Autodesk Inventor part; units mm, degrees
(part 2 of 3)
  spline S191 degree 2 poles (-31.6544, -13.3466) (-31.8311, -13.3678) (-32.0102, -13.4951) (-32.0102, -13.653) knots 0 0 0 1 2 2 2
  spline S192 degree 2 poles (-32.0102, -13.653) (-32.0102, -13.7684) (-31.8453, -13.9145) (-31.7063, -13.9145) knots 0 0 0 1 2 2 2
  spline S193 degree 2 poles (-31.7063, -13.9145) (-31.5178, -13.9145) (-31.2727, -13.6506) (-31.2727, -13.4503) knots 0 0 0 1 2 2 2
  line L231 (-31.2727, -13.4503) -> (-31.2727, -13.2925)
  spline S194 degree 2 poles (-29.3218, -12.7599) (-29.3948, -12.701) (-29.5362, -12.701) knots 0 0 0 1 1 1
  spline S195 degree 2 poles (-29.5362, -12.701) (-29.7176, -12.701) (-29.9627, -13.0309) (-29.9627, -13.3137) knots 0 0 0 1 2 2 2
  line L232 (-29.9627, -13.3137) -> (-29.9627, -14.1831)
  line L233 (-29.9627, -14.1831) -> (-30.3726, -14.1831)
  line L234 (-30.3726, -14.1831) -> (-30.3726, -12.3688)
  line L235 (-30.3726, -12.3688) -> (-29.9627, -12.3688)
  line L236 (-29.9627, -12.3688) -> (-29.9627, -12.7411)
  line L237 (-29.9627, -12.7411) -> (-29.9556, -12.7411)
  spline S196 degree 2 poles (-29.9556, -12.7411) (-29.8943, -12.5502) (-29.6446, -12.3358) (-29.4914, -12.3358) knots 0 0 0 1 2 2 2
  spline S197 degree 2 poles (-29.4914, -12.3358) (-29.3807, -12.3358) (-29.3218, -12.3688) knots 0 0 0 1 1 1
  line L238 (-29.3218, -12.3688) -> (-29.3218, -12.7599)
  line L239 (-28.6196, -14.1831) -> (-29.0296, -14.1831)
  line L240 (-29.0296, -14.1831) -> (-29.0296, -12.3688)
  line L241 (-29.0296, -12.3688) -> (-28.6196, -12.3688)
  line L242 (-28.6196, -12.3688) -> (-28.6196, -14.1831)
  spline S198 degree 2 poles (-28.8222, -11.9871) (-28.9236, -11.9871) (-29.0673, -11.8552) (-29.0673, -11.7538) knots 0 0 0 1 2 2 2
  spline S199 degree 2 poles (-29.0673, -11.7538) (-29.0673, -11.6525) (-28.9236, -11.5182) (-28.8222, -11.5182) knots 0 0 0 1 2 2 2
  spline S200 degree 2 poles (-28.8222, -11.5182) (-28.7186, -11.5182) (-28.5725, -11.6525) (-28.5725, -11.7538) knots 0 0 0 1 2 2 2
  spline S201 degree 2 poles (-28.5725, -11.7538) (-28.5725, -11.8504) (-28.7186, -11.9871) (-28.8222, -11.9871) knots 0 0 0 1 2 2 2
  line L243 (-27.6701, -14.1831) -> (-28.0824, -14.1831)
  line L244 (-28.0824, -14.1831) -> (-28.0824, -11.497)
  line L245 (-28.0824, -11.497) -> (-27.6701, -11.497)
  line L246 (-27.6701, -11.497) -> (-27.6701, -14.1831)
  line L247 (-26.7229, -14.1831) -> (-27.1352, -14.1831)
  line L248 (-27.1352, -14.1831) -> (-27.1352, -11.497)
  line L249 (-27.1352, -11.497) -> (-26.7229, -11.497)
  line L250 (-26.7229, -11.497) -> (-26.7229, -14.1831)
  line L251 (-24.7955, -14.1831) -> (-25.196, -14.1831)
  line L252 (-25.196, -14.1831) -> (-25.196, -13.9004)
  line L253 (-25.196, -13.9004) -> (-25.2031, -13.9004)
  spline S202 degree 2 poles (-25.2031, -13.9004) (-25.3892, -14.2255) (-25.7521, -14.2255) knots 0 0 0 1 1 1
  spline S203 degree 2 poles (-25.7521, -14.2255) (-26.0207, -14.2255) (-26.3247, -13.9357) (-26.3247, -13.6954) knots 0 0 0 1 2 2 2
  spline S204 degree 2 poles (-26.3247, -13.6954) (-26.3247, -13.1817) (-25.7309, -13.0969) knots 0 0 0 1 1 1
  line L254 (-25.7309, -13.0969) -> (-25.1937, -13.0215)
  spline S205 degree 2 poles (-25.1937, -13.0215) (-25.1937, -12.6327) (-25.5612, -12.6327) knots 0 0 0 1 1 1
  spline S206 degree 2 poles (-25.5612, -12.6327) (-25.8864, -12.6327) (-26.1456, -12.8566) knots 0 0 0 1 1 1
  line L255 (-26.1456, -12.8566) -> (-26.1456, -12.496)
  spline S207 degree 2 poles (-26.1456, -12.496) (-25.8605, -12.3264) (-25.4835, -12.3264) knots 0 0 0 1 1 1
  spline S208 degree 2 poles (-25.4835, -12.3264) (-24.7955, -12.3264) (-24.7955, -13.0026) knots 0 0 0 1 1 1
  line L256 (-24.7955, -13.0026) -> (-24.7955, -14.1831)
  line L257 (-25.1937, -13.2925) -> (-25.5754, -13.3466)
  spline S209 degree 2 poles (-25.5754, -13.3466) (-25.7521, -13.3678) (-25.9312, -13.4951) (-25.9312, -13.653) knots 0 0 0 1 2 2 2
  spline S210 degree 2 poles (-25.9312, -13.653) (-25.9312, -13.7684) (-25.7662, -13.9145) (-25.6272, -13.9145) knots 0 0 0 1 2 2 2
  spline S211 degree 2 poles (-25.6272, -13.9145) (-25.4387, -13.9145) (-25.1937, -13.6506) (-25.1937, -13.4503) knots 0 0 0 1 2 2 2
  line L258 (-25.1937, -13.4503) -> (-25.1937, -13.2925)
  line L259 (-21.8266, -14.1831) -> (-23.2522, -14.1831)
  line L260 (-23.2522, -14.1831) -> (-23.2522, -11.6431)
  line L261 (-23.2522, -11.6431) -> (-21.8832, -11.6431)
  line L262 (-21.8832, -11.6431) -> (-21.8832, -12.0012)
  line L263 (-21.8832, -12.0012) -> (-22.8304, -12.0012)
  line L264 (-22.8304, -12.0012) -> (-22.8304, -12.7199)
  line L265 (-22.8304, -12.7199) -> (-21.9562, -12.7199)
  line L266 (-21.9562, -12.7199) -> (-21.9562, -13.0757)
  line L267 (-21.9562, -13.0757) -> (-22.8304, -13.0757)
  line L268 (-22.8304, -13.0757) -> (-22.8304, -13.8273)
  line L269 (-22.8304, -13.8273) -> (-21.8266, -13.8273)
  line L270 (-21.8266, -13.8273) -> (-21.8266, -14.1831)
  line L271 (-21.5345, -14.1266) -> (-21.5345, -13.7472)
  spline S212 degree 2 poles (-21.5345, -13.7472) (-21.3036, -13.9216) (-21.0255, -13.9216) knots 0 0 0 1 1 1
  spline S213 degree 2 poles (-21.0255, -13.9216) (-20.6532, -13.9216) (-20.6532, -13.7001) knots 0 0 0 1 1 1
  spline S214 degree 2 poles (-20.6532, -13.7001) (-20.6532, -13.6388) (-20.7169, -13.5516) (-20.8252, -13.4857) (-20.9713, -13.4315) (-21.0632, -13.3985) knots 0 0 0 1 2 3 4 4 4
  spline S215 degree 2 poles (-21.0632, -13.3985) (-21.174, -13.3537) (-21.353, -13.2548) (-21.4709, -13.1299) (-21.5321, -12.9696) (-21.5321, -12.8636) knots 0 0 0 1 2 3 4 4 4
  spline S216 degree 2 poles (-21.5321, -12.8636) (-21.5321, -12.7317) (-21.4072, -12.5314) (-21.1975, -12.3947) (-20.9336, -12.3264) (-20.7923, -12.3264) knots 0 0 0 1 2 3 4 4 4
  spline S217 degree 2 poles (-20.7923, -12.3264) (-20.5401, -12.3264) (-20.3422, -12.4018) knots 0 0 0 1 1 1
  line L272 (-20.3422, -12.4018) -> (-20.3422, -12.7623)
  spline S218 degree 2 poles (-20.3422, -12.7623) (-20.5331, -12.6304) (-20.7805, -12.6304) knots 0 0 0 1 1 1
  spline S219 degree 2 poles (-20.7805, -12.6304) (-20.8582, -12.6304) (-20.9831, -12.6633) (-21.0727, -12.7199) (-21.1221, -12.8) (-21.1221, -12.8471) knots 0 0 0 1 2 3 4 4 4
  spline S220 degree 2 poles (-21.1221, -12.8471) (-21.1221, -12.906) (-21.0727, -12.9861) (-20.976, -13.0498) (-20.8394, -13.1016) (-20.7499, -13.1299) knots 0 0 0 1 2 3 4 4 4
  spline S221 degree 2 poles (-20.7499, -13.1299) (-20.6344, -13.1794) (-20.4483, -13.2783) (-20.3163, -13.4032) (-20.2456, -13.5681) (-20.2456, -13.6812) knots 0 0 0 1 2 3 4 4 4
  spline S222 degree 2 poles (-20.2456, -13.6812) (-20.2456, -13.8202) (-20.3729, -14.0252) (-20.5849, -14.1595) (-20.8629, -14.2255) (-21.0185, -14.2255) knots 0 0 0 1 2 3 4 4 4
  spline S223 degree 2 poles (-21.0185, -14.2255) (-21.3153, -14.2255) (-21.5345, -14.1266) knots 0 0 0 1 1 1
  spline S224 degree 2 poles (-18.8979, -14.1619) (-19.0204, -14.2232) (-19.216, -14.2232) knots 0 0 0 1 1 1
  spline S225 degree 2 poles (-19.216, -14.2232) (-19.7437, -14.2232) (-19.7437, -13.7166) knots 0 0 0 1 1 1
  line L273 (-19.7437, -13.7166) -> (-19.7437, -12.6916)
  line L274 (-19.7437, -12.6916) -> (-20.0477, -12.6916)
  line L275 (-20.0477, -12.6916) -> (-20.0477, -12.3688)
  line L276 (-20.0477, -12.3688) -> (-19.7437, -12.3688)
  line L277 (-19.7437, -12.3688) -> (-19.7437, -11.9494)
  line L278 (-19.7437, -11.9494) -> (-19.3338, -11.8316)
  line L279 (-19.3338, -11.8316) -> (-19.3338, -12.3688)
  line L280 (-19.3338, -12.3688) -> (-18.8979, -12.3688)
  line L281 (-18.8979, -12.3688) -> (-18.8979, -12.6916)
  line L282 (-18.8979, -12.6916) -> (-19.3338, -12.6916)
  line L283 (-19.3338, -12.6916) -> (-19.3338, -13.5988)
  spline S226 degree 2 poles (-19.3338, -13.5988) (-19.3338, -13.759) (-19.216, -13.898) (-19.0793, -13.898) knots 0 0 0 1 2 2 2
  spline S227 degree 2 poles (-19.0793, -13.898) (-18.9756, -13.898) (-18.8979, -13.8367) knots 0 0 0 1 1 1
  line L284 (-18.8979, -13.8367) -> (-18.8979, -14.1619)
  line L285 (-18.1345, -14.1831) -> (-18.5444, -14.1831)
  line L286 (-18.5444, -14.1831) -> (-18.5444, -12.3688)
  line L287 (-18.5444, -12.3688) -> (-18.1345, -12.3688)
  line L288 (-18.1345, -12.3688) -> (-18.1345, -14.1831)
  spline S228 degree 2 poles (-18.3371, -11.9871) (-18.4384, -11.9871) (-18.5821, -11.8552) (-18.5821, -11.7538) knots 0 0 0 1 2 2 2
  spline S229 degree 2 poles (-18.5821, -11.7538) (-18.5821, -11.6525) (-18.4384, -11.5182) (-18.3371, -11.5182) knots 0 0 0 1 2 2 2
  spline S230 degree 2 poles (-18.3371, -11.5182) (-18.2334, -11.5182) (-18.0873, -11.6525) (-18.0873, -11.7538) knots 0 0 0 1 2 2 2
  spline S231 degree 2 poles (-18.0873, -11.7538) (-18.0873, -11.8504) (-18.2334, -11.9871) (-18.3371, -11.9871) knots 0 0 0 1 2 2 2
  line L289 (-14.8852, -14.1831) -> (-15.2952, -14.1831)
  line L290 (-15.2952, -14.1831) -> (-15.2952, -13.1935)
  spline S232 degree 2 poles (-15.2952, -13.1935) (-15.2952, -12.9084) (-15.4578, -12.6539) (-15.6486, -12.6539) knots 0 0 0 1 2 2 2
  spline S233 degree 2 poles (-15.6486, -12.6539) (-15.8089, -12.6539) (-16.0351, -12.9767) (-16.0351, -13.2006) knots 0 0 0 1 2 2 2
  line L291 (-16.0351, -13.2006) -> (-16.0351, -14.1831)
  line L292 (-16.0351, -14.1831) -> (-16.4474, -14.1831)
  line L293 (-16.4474, -14.1831) -> (-16.4474, -13.1605)
  spline S234 degree 2 poles (-16.4474, -13.1605) (-16.4474, -12.6539) (-16.8055, -12.6539) knots 0 0 0 1 1 1
  spline S235 degree 2 poles (-16.8055, -12.6539) (-16.9728, -12.6539) (-17.1873, -12.9579) (-17.1873, -13.2006) knots 0 0 0 1 2 2 2
  line L294 (-17.1873, -13.2006) -> (-17.1873, -14.1831)
  line L295 (-17.1873, -14.1831) -> (-17.5972, -14.1831)
  line L296 (-17.5972, -14.1831) -> (-17.5972, -12.3688)
  line L297 (-17.5972, -12.3688) -> (-17.1873, -12.3688)
  line L298 (-17.1873, -12.3688) -> (-17.1873, -12.6563)
  line L299 (-17.1873, -12.6563) -> (-17.1802, -12.6563)
  spline S236 degree 2 poles (-17.1802, -12.6563) (-16.9823, -12.3264) (-16.6076, -12.3264) knots 0 0 0 1 1 1
  spline S237 degree 2 poles (-16.6076, -12.3264) (-16.4191, -12.3264) (-16.1387, -12.5337) (-16.0869, -12.701) knots 0 0 0 1 2 2 2
  spline S238 degree 2 poles (-16.0869, -12.701) (-15.8843, -12.3264) (-15.4837, -12.3264) knots 0 0 0 1 1 1
  spline S239 degree 2 poles (-15.4837, -12.3264) (-14.8852, -12.3264) (-14.8852, -13.0663) knots 0 0 0 1 1 1
  line L300 (-14.8852, -13.0663) -> (-14.8852, -14.1831)
  line L301 (-12.8023, -14.1831) -> (-13.2123, -14.1831)
  line L302 (-13.2123, -14.1831) -> (-13.2123, -13.8956)
  line L303 (-13.2123, -13.8956) -> (-13.2194, -13.8956)
  spline S240 degree 2 poles (-13.2194, -13.8956) (-13.3985, -14.2255) (-13.7778, -14.2255) knots 0 0 0 1 1 1
  spline S241 degree 2 poles (-13.7778, -14.2255) (-14.4187, -14.2255) (-14.4187, -13.4527) knots 0 0 0 1 1 1
  line L304 (-14.4187, -13.4527) -> (-14.4187, -12.3688)
  line L305 (-14.4187, -12.3688) -> (-14.0087, -12.3688)
  line L306 (-14.0087, -12.3688) -> (-14.0087, -13.4103)
  spline S242 degree 2 poles (-14.0087, -13.4103) (-14.0087, -13.9004) (-13.6317, -13.9004) knots 0 0 0 1 1 1
  spline S243 degree 2 poles (-13.6317, -13.9004) (-13.4479, -13.9004) (-13.2123, -13.6317) (-13.2123, -13.4126) knots 0 0 0 1 2 2 2
  line L307 (-13.2123, -13.4126) -> (-13.2123, -12.3688)
  line L308 (-13.2123, -12.3688) -> (-12.8023, -12.3688)
  line L309 (-12.8023, -12.3688) -> (-12.8023, -14.1831)
  line L310 (-11.8528, -14.1831) -> (-12.2651, -14.1831)
  line L311 (-12.2651, -14.1831) -> (-12.2651, -11.497)
  line L312 (-12.2651, -11.497) -> (-11.8528, -11.497)
  line L313 (-11.8528, -11.497) -> (-11.8528, -14.1831)
  line L314 (-9.9254, -14.1831) -> (-10.326, -14.1831)
  line L315 (-10.326, -14.1831) -> (-10.326, -13.9004)
  line L316 (-10.326, -13.9004) -> (-10.333, -13.9004)
  spline S244 degree 2 poles (-10.333, -13.9004) (-10.5192, -14.2255) (-10.882, -14.2255) knots 0 0 0 1 1 1
  spline S245 degree 2 poles (-10.882, -14.2255) (-11.1506, -14.2255) (-11.4546, -13.9357) (-11.4546, -13.6954) knots 0 0 0 1 2 2 2
  spline S246 degree 2 poles (-11.4546, -13.6954) (-11.4546, -13.1817) (-10.8608, -13.0969) knots 0 0 0 1 1 1
  line L317 (-10.8608, -13.0969) -> (-10.3236, -13.0215)
  spline S247 degree 2 poles (-10.3236, -13.0215) (-10.3236, -12.6327) (-10.6912, -12.6327) knots 0 0 0 1 1 1
  spline S248 degree 2 poles (-10.6912, -12.6327) (-11.0163, -12.6327) (-11.2755, -12.8566) knots 0 0 0 1 1 1
  line L318 (-11.2755, -12.8566) -> (-11.2755, -12.496)
  spline S249 degree 2 poles (-11.2755, -12.496) (-10.9904, -12.3264) (-10.6134, -12.3264) knots 0 0 0 1 1 1
  spline S250 degree 2 poles (-10.6134, -12.3264) (-9.9254, -12.3264) (-9.9254, -13.0026) knots 0 0 0 1 1 1
  line L319 (-9.9254, -13.0026) -> (-9.9254, -14.1831)
  line L320 (-10.3236, -13.2925) -> (-10.7053, -13.3466)
  spline S251 degree 2 poles (-10.7053, -13.3466) (-10.882, -13.3678) (-11.0611, -13.4951) (-11.0611, -13.653) knots 0 0 0 1 2 2 2
  spline S252 degree 2 poles (-11.0611, -13.653) (-11.0611, -13.7684) (-10.8962, -13.9145) (-10.7571, -13.9145) knots 0 0 0 1 2 2 2
  spline S253 degree 2 poles (-10.7571, -13.9145) (-10.5686, -13.9145) (-10.3236, -13.6506) (-10.3236, -13.4503) knots 0 0 0 1 2 2 2
  line L321 (-10.3236, -13.4503) -> (-10.3236, -13.2925)
  line L322 (-7.7742, -14.1831) -> (-8.1865, -14.1831)
  line L323 (-8.1865, -14.1831) -> (-8.1865, -13.8744)
  line L324 (-8.1865, -13.8744) -> (-8.1936, -13.8744)
  spline S254 degree 2 poles (-8.1936, -13.8744) (-8.3915, -14.2255) (-8.8038, -14.2255) knots 0 0 0 1 1 1
  spline S255 degree 2 poles (-8.8038, -14.2255) (-9.1384, -14.2255) (-9.5413, -13.7378) (-9.5413, -13.3184) knots 0 0 0 1 2 2 2
  spline S256 degree 2 poles (-9.5413, -13.3184) (-9.5413, -12.8683) (-9.096, -12.3264) (-8.7261, -12.3264) knots 0 0 0 1 2 2 2
  spline S257 degree 2 poles (-8.7261, -12.3264) (-8.3609, -12.3264) (-8.1936, -12.6209) knots 0 0 0 1 1 1
  line L325 (-8.1936, -12.6209) -> (-8.1865, -12.6209)
  line L326 (-8.1865, -12.6209) -> (-8.1865, -11.497)
  line L327 (-8.1865, -11.497) -> (-7.7742, -11.497)
  line L328 (-7.7742, -11.497) -> (-7.7742, -14.1831)
  line L329 (-8.1818, -13.3537) -> (-8.1818, -13.1157)
  spline S258 degree 2 poles (-8.1818, -13.1157) (-8.1818, -12.9225) (-8.4316, -12.6539) (-8.6271, -12.6539) knots 0 0 0 1 2 2 2
  spline S259 degree 2 poles (-8.6271, -12.6539) (-8.858, -12.6539) (-9.1219, -12.9979) (-9.1219, -13.3019) knots 0 0 0 1 2 2 2
  spline S260 degree 2 poles (-9.1219, -13.3019) (-9.1219, -13.5799) (-8.8675, -13.9004) (-8.653, -13.9004) knots 0 0 0 1 2 2 2
  spline S261 degree 2 poles (-8.653, -13.9004) (-8.4433, -13.9004) (-8.1818, -13.5893) (-8.1818, -13.3537) knots 0 0 0 1 2 2 2
  spline S262 degree 2 poles (-6.4335, -14.2255) (-6.8529, -14.2255) (-7.3548, -13.7166) (-7.3548, -13.2972) knots 0 0 0 1 2 2 2
  spline S263 degree 2 poles (-7.3548, -13.2972) (-7.3548, -12.8401) (-6.8317, -12.3264) (-6.3887, -12.3264) knots 0 0 0 1 2 2 2
  spline S264 degree 2 poles (-6.3887, -12.3264) (-5.9646, -12.3264) (-5.4886, -12.8259) (-5.4886, -13.2689) knots 0 0 0 1 2 2 2
  spline S265 degree 2 poles (-5.4886, -13.2689) (-5.4886, -13.7024) (-6.0023, -14.2255) (-6.4335, -14.2255) knots 0 0 0 1 2 2 2
  spline S266 degree 2 poles (-6.4146, -12.6539) (-6.655, -12.6539) (-6.9354, -12.9909) (-6.9354, -13.2877) knots 0 0 0 1 2 2 2
  spline S267 degree 2 poles (-6.9354, -13.2877) (-6.9354, -13.5728) (-6.6526, -13.9004) (-6.4146, -13.9004) knots 0 0 0 1 2 2 2
  spline S268 degree 2 poles (-6.4146, -13.9004) (-6.1719, -13.9004) (-5.9104, -13.5776) (-5.9104, -13.2807) knots 0 0 0 1 2 2 2
  spline S269 degree 2 poles (-5.9104, -13.2807) (-5.9104, -12.9791) (-6.1719, -12.6539) (-6.4146, -12.6539) knots 0 0 0 1 2 2 2
  spline S270 degree 2 poles (-4.0184, -12.7599) (-4.0914, -12.701) (-4.2328, -12.701) knots 0 0 0 1 1 1
  spline S271 degree 2 poles (-4.2328, -12.701) (-4.4142, -12.701) (-4.6593, -13.0309) (-4.6593, -13.3137) knots 0 0 0 1 2 2 2
  line L330 (-4.6593, -13.3137) -> (-4.6593, -14.1831)
  line L331 (-4.6593, -14.1831) -> (-5.0692, -14.1831)
  line L332 (-5.0692, -14.1831) -> (-5.0692, -12.3688)
  line L333 (-5.0692, -12.3688) -> (-4.6593, -12.3688)
  line L334 (-4.6593, -12.3688) -> (-4.6593, -12.7411)
  line L335 (-4.6593, -12.7411) -> (-4.6522, -12.7411)
  spline S272 degree 2 poles (-4.6522, -12.7411) (-4.5909, -12.5502) (-4.3412, -12.3358) (-4.188, -12.3358) knots 0 0 0 1 2 2 2
  spline S273 degree 2 poles (-4.188, -12.3358) (-4.0773, -12.3358) (-4.0184, -12.3688) knots 0 0 0 1 1 1
  line L336 (-4.0184, -12.3688) -> (-4.0184, -12.7599)
  line L337 (-2.3337, -14.1831) -> (-2.7342, -14.1831)
  line L338 (-2.7342, -14.1831) -> (-2.7342, -13.9004)
  line L339 (-2.7342, -13.9004) -> (-2.7413, -13.9004)
  spline S274 degree 2 poles (-2.7413, -13.9004) (-2.9274, -14.2255) (-3.2903, -14.2255) knots 0 0 0 1 1 1
  spline S275 degree 2 poles (-3.2903, -14.2255) (-3.5589, -14.2255) (-3.8629, -13.9357) (-3.8629, -13.6954) knots 0 0 0 1 2 2 2
  spline S276 degree 2 poles (-3.8629, -13.6954) (-3.8629, -13.1817) (-3.2691, -13.0969) knots 0 0 0 1 1 1
  line L340 (-3.2691, -13.0969) -> (-2.7319, -13.0215)
  spline S277 degree 2 poles (-2.7319, -13.0215) (-2.7319, -12.6327) (-3.0994, -12.6327) knots 0 0 0 1 1 1
  spline S278 degree 2 poles (-3.0994, -12.6327) (-3.4246, -12.6327) (-3.6838, -12.8566) knots 0 0 0 1 1 1
  line L341 (-3.6838, -12.8566) -> (-3.6838, -12.496)
  spline S279 degree 2 poles (-3.6838, -12.496) (-3.3987, -12.3264) (-3.0217, -12.3264) knots 0 0 0 1 1 1
  spline S280 degree 2 poles (-3.0217, -12.3264) (-2.3337, -12.3264) (-2.3337, -13.0026) knots 0 0 0 1 1 1
  line L342 (-2.3337, -13.0026) -> (-2.3337, -14.1831)
  line L343 (-2.7319, -13.2925) -> (-3.1136, -13.3466)
  spline S281 degree 2 poles (-3.1136, -13.3466) (-3.2903, -13.3678) (-3.4694, -13.4951) (-3.4694, -13.653) knots 0 0 0 1 2 2 2
  spline S282 degree 2 poles (-3.4694, -13.653) (-3.4694, -13.7684) (-3.3044, -13.9145) (-3.1654, -13.9145) knots 0 0 0 1 2 2 2
  spline S283 degree 2 poles (-3.1654, -13.9145) (-2.9769, -13.9145) (-2.7319, -13.6506) (-2.7319, -13.4503) knots 0 0 0 1 2 2 2
  line L344 (-2.7319, -13.4503) -> (-2.7319, -13.2925)
  line L345 (1.2007, -11.6431) -> (0.2888, -14.1831)
  line L346 (0.2888, -14.1831) -> (-0.1824, -14.1831)
  line L347 (-0.1824, -14.1831) -> (-1.0778, -11.6431)
  line L348 (-1.0778, -11.6431) -> (-0.6183, -11.6431)
  line L349 (-0.6183, -11.6431) -> (0.0084, -13.5705)
  spline S284 degree 2 poles (0.0084, -13.5705) (0.039, -13.6624) (0.0555, -13.7849) knots 0 0 0 1 1 1
  line L350 (0.0555, -13.7849) -> (0.0626, -13.7849)
  spline S285 degree 2 poles (0.0626, -13.7849) (0.0744, -13.6836) (0.1144, -13.5658) knots 0 0 0 1 1 1
  line L351 (0.1144, -13.5658) -> (0.7553, -11.6431)
  line L352 (0.7553, -11.6431) -> (1.2007, -11.6431)
  line L353 (3.6912, -14.1831) -> (3.2317, -14.1831)
  line L354 (3.2317, -14.1831) -> (2.0183, -12.317)
  spline S286 degree 2 poles (2.0183, -12.317) (1.9711, -12.2463) (1.9429, -12.1685) knots 0 0 0 1 1 1
  line L355 (1.9429, -12.1685) -> (1.9311, -12.1685)
  spline S287 degree 2 poles (1.9311, -12.1685) (1.9452, -12.251) (1.9452, -12.5173) knots 0 0 0 1 1 1
  line L356 (1.9452, -12.5173) -> (1.9452, -14.1831)
  line L357 (1.9452, -14.1831) -> (1.5376, -14.1831)
  line L358 (1.5376, -14.1831) -> (1.5376, -11.6431)
  line L359 (1.5376, -11.6431) -> (2.0277, -11.6431)
  line L360 (2.0277, -11.6431) -> (3.2011, -13.4668)
  spline S288 degree 2 poles (3.2011, -13.4668) (3.2765, -13.5799) (3.2977, -13.6223) knots 0 0 0 1 1 1
  line L361 (3.2977, -13.6223) -> (3.3048, -13.6223)
  spline S289 degree 2 poles (3.3048, -13.6223) (3.2859, -13.521) (3.2859, -13.2807) knots 0 0 0 1 1 1
  line L362 (3.2859, -13.2807) -> (3.2859, -11.6431)
  line L363 (3.2859, -11.6431) -> (3.6912, -11.6431)
  line L364 (3.6912, -11.6431) -> (3.6912, -14.1831)
  line L365 (4.2025, -14.0818) -> (4.2025, -13.6482)
  spline S290 degree 2 poles (4.2025, -13.6482) (4.2614, -13.7024) (4.424, -13.7873) (4.603, -13.8438) (4.7845, -13.8768) (4.8599, -13.8768) knots 0 0 0 1 2 3 4 4 4
  spline S291 degree 2 poles (4.8599, -13.8768) (5.1261, -13.8768) (5.3876, -13.7001) (5.3876, -13.5304) knots 0 0 0 1 2 2 2
  spline S292 degree 2 poles (5.3876, -13.5304) (5.3876, -13.4409) (5.3005, -13.3089) (5.145, -13.1982) (4.9329, -13.0969) (4.8127, -13.0427) knots 0 0 0 1 2 3 4 4 4
  spline S293 degree 2 poles (4.8127, -13.0427) (4.6831, -12.9744) (4.4617, -12.8306) (4.2967, -12.661) (4.2025, -12.4442) (4.2025, -12.2981) knots 0 0 0 1 2 3 4 4 4
  spline S294 degree 2 poles (4.2025, -12.2981) (4.2025, -12.1191) (4.3627, -11.8552) (4.6266, -11.6832) (4.9635, -11.6007) (5.1402, -11.6007) knots 0 0 0 1 2 3 4 4 4
  spline S295 degree 2 poles (5.1402, -11.6007) (5.5384, -11.6007) (5.7199, -11.6902) knots 0 0 0 1 1 1
  line L366 (5.7199, -11.6902) -> (5.7199, -12.1073)
  spline S296 degree 2 poles (5.7199, -12.1073) (5.5031, -11.9518) (5.1638, -11.9518) knots 0 0 0 1 1 1
  spline S297 degree 2 poles (5.1638, -11.9518) (5.0696, -11.9518) (4.8834, -11.9871) (4.7373, -12.0696) (4.6454, -12.1968) (4.6454, -12.2863) knots 0 0 0 1 2 3 4 4 4
  spline S298 degree 2 poles (4.6454, -12.2863) (4.6454, -12.3712) (4.7161, -12.496) (4.8528, -12.5974) (5.0484, -12.6963) (5.1779, -12.7529) knots 0 0 0 1 2 3 4 4 4
  spline S299 degree 2 poles (5.1779, -12.7529) (5.3099, -12.8212) (5.5455, -12.9744) (5.7246, -13.1581) (5.8306, -13.382) (5.8306, -13.5257) knots 0 0 0 1 2 3 4 4 4
  spline S300 degree 2 poles (5.8306, -13.5257) (5.8306, -13.7189) (5.6751, -13.9852) (5.4112, -14.1501) (5.0672, -14.2255) (4.874, -14.2255) knots 0 0 0 1 2 3 4 4 4
  spline S301 degree 2 poles (4.874, -14.2255) (4.8104, -14.2255) (4.6242, -14.2067) (4.431, -14.169) (4.2567, -14.1148) (4.2025, -14.0818) knots 0 0 0 1 2 3 4 4 4
  line L367 (-26.4967, -19.0566) -> (-26.9891, -19.0566)
  line L368 (-26.9891, -19.0566) -> (-27.3944, -18.3757)
  spline S302 degree 2 poles (-27.3944, -18.3757) (-27.4486, -18.2814) (-27.5546, -18.1495) (-27.663, -18.0647) (-27.7902, -18.0246) (-27.868, -18.0246) knots 0 0 0 1 2 3 4 4 4
  line L369 (-27.868, -18.0246) -> (-28.04, -18.0246)
  line L370 (-28.04, -18.0246) -> (-28.04, -19.0566)
  line L371 (-28.04, -19.0566) -> (-28.4594, -19.0566)
  line L372 (-28.4594, -19.0566) -> (-28.4594, -16.5166)
  line L373 (-28.4594, -16.5166) -> (-27.6229, -16.5166)
  spline S303 degree 2 poles (-27.6229, -16.5166) (-27.4439, -16.5166) (-27.1423, -16.6015) (-26.9184, -16.7735) (-26.7935, -17.0303) (-26.7935, -17.2023) knots 0 0 0 1 2 3 4 4 4
  spline S304 degree 2 poles (-26.7935, -17.2023) (-26.7935, -17.3366) (-26.8737, -17.5604) (-27.0197, -17.7372) (-27.2271, -17.8597) (-27.3567, -17.8927) knots 0 0 0 1 2 3 4 4 4
  line L374 (-27.3567, -17.8927) -> (-27.3567, -17.8997)
  spline S305 degree 2 poles (-27.3567, -17.8997) (-27.2883, -17.9398) (-27.1847, -18.034) (-27.0928, -18.133) (-27.0032, -18.2579) (-26.9467, -18.3427) knots 0 0 0 1 2 3 4 4 4
  line L375 (-26.9467, -18.3427) -> (-26.4967, -19.0566)
  line L376 (-28.04, -16.8583) -> (-28.04, -17.683)
  line L377 (-28.04, -17.683) -> (-27.6889, -17.683)
  spline S306 degree 2 poles (-27.6889, -17.683) (-27.5899, -17.683) (-27.4274, -17.6217) (-27.3048, -17.5086) (-27.2389, -17.346) (-27.2389, -17.2447) knots 0 0 0 1 2 3 4 4 4
  spline S307 degree 2 poles (-27.2389, -17.2447) (-27.2389, -17.0633) (-27.4698, -16.8583) (-27.6842, -16.8583) knots 0 0 0 1 2 2 2
  line L378 (-27.6842, -16.8583) -> (-28.04, -16.8583)
  spline S308 degree 2 poles (-25.4411, -19.0991) (-25.8605, -19.0991) (-26.3624, -18.5901) (-26.3624, -18.1707) knots 0 0 0 1 2 2 2
  spline S309 degree 2 poles (-26.3624, -18.1707) (-26.3624, -17.7136) (-25.8393, -17.1999) (-25.3963, -17.1999) knots 0 0 0 1 2 2 2
  spline S310 degree 2 poles (-25.3963, -17.1999) (-24.9722, -17.1999) (-24.4962, -17.6995) (-24.4962, -18.1424) knots 0 0 0 1 2 2 2
  spline S311 degree 2 poles (-24.4962, -18.1424) (-24.4962, -18.576) (-25.0099, -19.0991) (-25.4411, -19.0991) knots 0 0 0 1 2 2 2
  spline S312 degree 2 poles (-25.4222, -17.5275) (-25.6626, -17.5275) (-25.9429, -17.8644) (-25.9429, -18.1613) knots 0 0 0 1 2 2 2
  spline S313 degree 2 poles (-25.9429, -18.1613) (-25.9429, -18.4464) (-25.6602, -18.7739) (-25.4222, -18.7739) knots 0 0 0 1 2 2 2
  spline S314 degree 2 poles (-25.4222, -18.7739) (-25.1795, -18.7739) (-24.918, -18.4511) (-24.918, -18.1542) knots 0 0 0 1 2 2 2
  spline S315 degree 2 poles (-24.918, -18.1542) (-24.918, -17.8526) (-25.1795, -17.5275) (-25.4222, -17.5275) knots 0 0 0 1 2 2 2
  line L379 (-22.4275, -19.0566) -> (-22.8398, -19.0566)
  line L380 (-22.8398, -19.0566) -> (-22.8398, -18.748)
  line L381 (-22.8398, -18.748) -> (-22.8469, -18.748)
  spline S316 degree 2 poles (-22.8469, -18.748) (-23.0448, -19.0991) (-23.4571, -19.0991) knots 0 0 0 1 1 1
  spline S317 degree 2 poles (-23.4571, -19.0991) (-23.7917, -19.0991) (-24.1946, -18.6113) (-24.1946, -18.1919) knots 0 0 0 1 2 2 2
  spline S318 degree 2 poles (-24.1946, -18.1919) (-24.1946, -17.7419) (-23.7493, -17.1999) (-23.3794, -17.1999) knots 0 0 0 1 2 2 2
  spline S319 degree 2 poles (-23.3794, -17.1999) (-23.0142, -17.1999) (-22.8469, -17.4945) knots 0 0 0 1 1 1
  line L382 (-22.8469, -17.4945) -> (-22.8398, -17.4945)
  line L383 (-22.8398, -17.4945) -> (-22.8398, -16.3706)
  line L384 (-22.8398, -16.3706) -> (-22.4275, -16.3706)
  line L385 (-22.4275, -16.3706) -> (-22.4275, -19.0566)
  line L386 (-22.8351, -18.2273) -> (-22.8351, -17.9893)
  spline S320 degree 2 poles (-22.8351, -17.9893) (-22.8351, -17.7961) (-23.0849, -17.5275) (-23.2804, -17.5275) knots 0 0 0 1 2 2 2
  spline S321 degree 2 poles (-23.2804, -17.5275) (-23.5113, -17.5275) (-23.7752, -17.8715) (-23.7752, -18.1754) knots 0 0 0 1 2 2 2
  spline S322 degree 2 poles (-23.7752, -18.1754) (-23.7752, -18.4535) (-23.5208, -18.7739) (-23.3063, -18.7739) knots 0 0 0 1 2 2 2
  spline S323 degree 2 poles (-23.3063, -18.7739) (-23.0966, -18.7739) (-22.8351, -18.4629) (-22.8351, -18.2273) knots 0 0 0 1 2 2 2
  spline S324 degree 2 poles (-20.8394, -17.6335) (-20.9124, -17.5746) (-21.0538, -17.5746) knots 0 0 0 1 1 1
  spline S325 degree 2 poles (-21.0538, -17.5746) (-21.2352, -17.5746) (-21.4803, -17.9045) (-21.4803, -18.1872) knots 0 0 0 1 2 2 2
  line L387 (-21.4803, -18.1872) -> (-21.4803, -19.0566)
  line L388 (-21.4803, -19.0566) -> (-21.8903, -19.0566)
  line L389 (-21.8903, -19.0566) -> (-21.8903, -17.2424)
  line L390 (-21.8903, -17.2424) -> (-21.4803, -17.2424)
  line L391 (-21.4803, -17.2424) -> (-21.4803, -17.6146)
  line L392 (-21.4803, -17.6146) -> (-21.4732, -17.6146)
  spline S326 degree 2 poles (-21.4732, -17.6146) (-21.4119, -17.4238) (-21.1622, -17.2094) (-21.009, -17.2094) knots 0 0 0 1 2 2 2
  spline S327 degree 2 poles (-21.009, -17.2094) (-20.8983, -17.2094) (-20.8394, -17.2424) knots 0 0 0 1 1 1
  line L393 (-20.8394, -17.2424) -> (-20.8394, -17.6335)
  line L394 (-20.1372, -19.0566) -> (-20.5472, -19.0566)
  line L395 (-20.5472, -19.0566) -> (-20.5472, -17.2424)
  line L396 (-20.5472, -17.2424) -> (-20.1372, -17.2424)
  line L397 (-20.1372, -17.2424) -> (-20.1372, -19.0566)
  spline S328 degree 2 poles (-20.3399, -16.8606) (-20.4412, -16.8606) (-20.5849, -16.7287) (-20.5849, -16.6274) knots 0 0 0 1 2 2 2
  spline S329 degree 2 poles (-20.5849, -16.6274) (-20.5849, -16.5261) (-20.4412, -16.3918) (-20.3399, -16.3918) knots 0 0 0 1 2 2 2
  spline S330 degree 2 poles (-20.3399, -16.3918) (-20.2362, -16.3918) (-20.0901, -16.5261) (-20.0901, -16.6274) knots 0 0 0 1 2 2 2
  spline S331 degree 2 poles (-20.0901, -16.6274) (-20.0901, -16.724) (-20.2362, -16.8606) (-20.3399, -16.8606) knots 0 0 0 1 2 2 2
  spline S332 degree 2 poles (-17.9507, -18.9106) (-17.9507, -19.9096) (-18.9544, -19.9096) knots 0 0 0 1 1 1
  spline S333 degree 2 poles (-18.9544, -19.9096) (-19.3078, -19.9096) (-19.5717, -19.7918) knots 0 0 0 1 1 1
  line L398 (-19.5717, -19.7918) -> (-19.5717, -19.4148)
  spline S334 degree 2 poles (-19.5717, -19.4148) (-19.2749, -19.5844) (-19.0086, -19.5844) knots 0 0 0 1 1 1
  spline S335 degree 2 poles (-19.0086, -19.5844) (-18.3606, -19.5844) (-18.3606, -18.9506) knots 0 0 0 1 1 1
  line L399 (-18.3606, -18.9506) -> (-18.3606, -18.7527)
  line L400 (-18.3606, -18.7527) -> (-18.3677, -18.7527)
  spline S336 degree 2 poles (-18.3677, -18.7527) (-18.5727, -19.0991) (-18.9803, -19.0991) knots 0 0 0 1 1 1
  spline S337 degree 2 poles (-18.9803, -19.0991) (-19.3126, -19.0991) (-19.7178, -18.616) (-19.7178, -18.2084) knots 0 0 0 1 2 2 2
  spline S338 degree 2 poles (-19.7178, -18.2084) (-19.7178, -17.7466) (-19.2819, -17.1999) (-18.9002, -17.1999) knots 0 0 0 1 2 2 2
  spline S339 degree 2 poles (-18.9002, -17.1999) (-18.5421, -17.1999) (-18.3677, -17.4945) knots 0 0 0 1 1 1
  line L401 (-18.3677, -17.4945) -> (-18.3606, -17.4945)
  line L402 (-18.3606, -17.4945) -> (-18.3606, -17.2424)
  line L403 (-18.3606, -17.2424) -> (-17.9507, -17.2424)
  line L404 (-17.9507, -17.2424) -> (-17.9507, -18.9106)
  line L405 (-18.3583, -18.2249) -> (-18.3583, -17.9893)
  spline S340 degree 2 poles (-18.3583, -17.9893) (-18.3583, -17.7984) (-18.6104, -17.5275) (-18.8013, -17.5275) knots 0 0 0 1 2 2 2
  spline S341 degree 2 poles (-18.8013, -17.5275) (-19.0345, -17.5275) (-19.2984, -17.8738) (-19.2984, -18.1825) knots 0 0 0 1 2 2 2
  spline S342 degree 2 poles (-19.2984, -18.1825) (-19.2984, -18.4511) (-19.0439, -18.7715) (-18.8366, -18.7715) knots 0 0 0 1 2 2 2
  spline S343 degree 2 poles (-18.8366, -18.7715) (-18.6222, -18.7715) (-18.3583, -18.4652) (-18.3583, -18.2249) knots 0 0 0 1 2 2 2
  spline S344 degree 2 poles (-16.61, -19.0991) (-17.0294, -19.0991) (-17.5313, -18.5901) (-17.5313, -18.1707) knots 0 0 0 1 2 2 2
  spline S345 degree 2 poles (-17.5313, -18.1707) (-17.5313, -17.7136) (-17.0082, -17.1999) (-16.5652, -17.1999) knots 0 0 0 1 2 2 2
  spline S346 degree 2 poles (-16.5652, -17.1999) (-16.1411, -17.1999) (-15.6651, -17.6995) (-15.6651, -18.1424) knots 0 0 0 1 2 2 2
  spline S347 degree 2 poles (-15.6651, -18.1424) (-15.6651, -18.576) (-16.1788, -19.0991) (-16.61, -19.0991) knots 0 0 0 1 2 2 2
  spline S348 degree 2 poles (-16.5911, -17.5275) (-16.8315, -17.5275) (-17.1119, -17.8644) (-17.1119, -18.1613) knots 0 0 0 1 2 2 2
  spline S349 degree 2 poles (-17.1119, -18.1613) (-17.1119, -18.4464) (-16.8291, -18.7739) (-16.5911, -18.7739) knots 0 0 0 1 2 2 2
  spline S350 degree 2 poles (-16.5911, -18.7739) (-16.3484, -18.7739) (-16.0869, -18.4511) (-16.0869, -18.1542) knots 0 0 0 1 2 2 2
  spline S351 degree 2 poles (-16.0869, -18.1542) (-16.0869, -17.8526) (-16.3484, -17.5275) (-16.5911, -17.5275) knots 0 0 0 1 2 2 2
  line L406 (-12.833, -16.8748) -> (-13.7825, -16.8748)
  line L407 (-13.7825, -16.8748) -> (-13.7825, -17.6382)
  line L408 (-13.7825, -17.6382) -> (-12.906, -17.6382)
  line L409 (-12.906, -17.6382) -> (-12.906, -17.994)
  line L410 (-12.906, -17.994) -> (-13.7825, -17.994)
  line L411 (-13.7825, -17.994) -> (-13.7825, -19.0566)
  line L412 (-13.7825, -19.0566) -> (-14.2043, -19.0566)
  line L413 (-14.2043, -19.0566) -> (-14.2043, -16.5166)
  line L414 (-14.2043, -16.5166) -> (-12.833, -16.5166)
  line L415 (-12.833, -16.5166) -> (-12.833, -16.8748)
  line L416 (-12.0154, -19.0566) -> (-12.4253, -19.0566)
  line L417 (-12.4253, -19.0566) -> (-12.4253, -17.2424)
  line L418 (-12.4253, -17.2424) -> (-12.0154, -17.2424)
  line L419 (-12.0154, -17.2424) -> (-12.0154, -19.0566)
  spline S352 degree 2 poles (-12.218, -16.8606) (-12.3193, -16.8606) (-12.463, -16.7287) (-12.463, -16.6274) knots 0 0 0 1 2 2 2
  spline S353 degree 2 poles (-12.463, -16.6274) (-12.463, -16.5261) (-12.3193, -16.3918) (-12.218, -16.3918) knots 0 0 0 1 2 2 2
  spline S354 degree 2 poles (-12.218, -16.3918) (-12.1143, -16.3918) (-11.9682, -16.5261) (-11.9682, -16.6274) knots 0 0 0 1 2 2 2
  spline S355 degree 2 poles (-11.9682, -16.6274) (-11.9682, -16.724) (-12.1143, -16.8606) (-12.218, -16.8606) knots 0 0 0 1 2 2 2
  spline S356 degree 2 poles (-9.8288, -18.9106) (-9.8288, -19.9096) (-10.8325, -19.9096) knots 0 0 0 1 1 1
  spline S357 degree 2 poles (-10.8325, -19.9096) (-11.186, -19.9096) (-11.4499, -19.7918) knots 0 0 0 1 1 1
  line L420 (-11.4499, -19.7918) -> (-11.4499, -19.4148)
  spline S358 degree 2 poles (-11.4499, -19.4148) (-11.153, -19.5844) (-10.8867, -19.5844) knots 0 0 0 1 1 1
  spline S359 degree 2 poles (-10.8867, -19.5844) (-10.2388, -19.5844) (-10.2388, -18.9506) knots 0 0 0 1 1 1
  line L421 (-10.2388, -18.9506) -> (-10.2388, -18.7527)
  line L422 (-10.2388, -18.7527) -> (-10.2458, -18.7527)
  spline S360 degree 2 poles (-10.2458, -18.7527) (-10.4508, -19.0991) (-10.8585, -19.0991) knots 0 0 0 1 1 1
  spline S361 degree 2 poles (-10.8585, -19.0991) (-11.1907, -19.0991) (-11.596, -18.616) (-11.596, -18.2084) knots 0 0 0 1 2 2 2
  spline S362 degree 2 poles (-11.596, -18.2084) (-11.596, -17.7466) (-11.1601, -17.1999) (-10.7783, -17.1999) knots 0 0 0 1 2 2 2
  spline S363 degree 2 poles (-10.7783, -17.1999) (-10.4202, -17.1999) (-10.2458, -17.4945) knots 0 0 0 1 1 1
  line L423 (-10.2458, -17.4945) -> (-10.2388, -17.4945)
  line L424 (-10.2388, -17.4945) -> (-10.2388, -17.2424)
  line L425 (-10.2388, -17.2424) -> (-9.8288, -17.2424)
  line L426 (-9.8288, -17.2424) -> (-9.8288, -18.9106)
  line L427 (-10.2364, -18.2249) -> (-10.2364, -17.9893)
  spline S364 degree 2 poles (-10.2364, -17.9893) (-10.2364, -17.7984) (-10.4885, -17.5275) (-10.6794, -17.5275) knots 0 0 0 1 2 2 2
  spline S365 degree 2 poles (-10.6794, -17.5275) (-10.9127, -17.5275) (-11.1765, -17.8738) (-11.1765, -18.1825) knots 0 0 0 1 2 2 2
  spline S366 degree 2 poles (-11.1765, -18.1825) (-11.1765, -18.4511) (-10.9221, -18.7715) (-10.7147, -18.7715) knots 0 0 0 1 2 2 2
  spline S367 degree 2 poles (-10.7147, -18.7715) (-10.5003, -18.7715) (-10.2364, -18.4652) (-10.2364, -18.2249) knots 0 0 0 1 2 2 2
  line L428 (-7.7106, -19.0566) -> (-8.1205, -19.0566)
  line L429 (-8.1205, -19.0566) -> (-8.1205, -18.7692)
  line L430 (-8.1205, -18.7692) -> (-8.1276, -18.7692)
  spline S368 degree 2 poles (-8.1276, -18.7692) (-8.3067, -19.0991) (-8.686, -19.0991) knots 0 0 0 1 1 1
  spline S369 degree 2 poles (-8.686, -19.0991) (-9.3269, -19.0991) (-9.3269, -18.3262) knots 0 0 0 1 1 1
  line L431 (-9.3269, -18.3262) -> (-9.3269, -17.2424)
  line L432 (-9.3269, -17.2424) -> (-8.9169, -17.2424)
  line L433 (-8.9169, -17.2424) -> (-8.9169, -18.2838)
  spline S370 degree 2 poles (-8.9169, -18.2838) (-8.9169, -18.7739) (-8.5399, -18.7739) knots 0 0 0 1 1 1
  spline S371 degree 2 poles (-8.5399, -18.7739) (-8.3562, -18.7739) (-8.1205, -18.5053) (-8.1205, -18.2862) knots 0 0 0 1 2 2 2
  line L434 (-8.1205, -18.2862) -> (-8.1205, -17.2424)
  line L435 (-8.1205, -17.2424) -> (-7.7106, -17.2424)
  line L436 (-7.7106, -17.2424) -> (-7.7106, -19.0566)
  line L437 (-5.6394, -18.2602) -> (-6.8741, -18.2602)
  spline S372 degree 2 poles (-6.8741, -18.2602) (-6.867, -18.5124) (-6.5725, -18.7857) (-6.3133, -18.7857) knots 0 0 0 1 2 2 2
  spline S373 degree 2 poles (-6.3133, -18.7857) (-6.0235, -18.7857) (-5.7808, -18.6113) knots 0 0 0 1 1 1
  line L438 (-5.7808, -18.6113) -> (-5.7808, -18.9435)
  spline S374 degree 2 poles (-5.7808, -18.9435) (-6.0282, -19.0991) (-6.4358, -19.0991) knots 0 0 0 1 1 1
  spline S375 degree 2 poles (-6.4358, -19.0991) (-6.8364, -19.0991) (-7.2911, -18.6042) (-7.2911, -18.1566) knots 0 0 0 1 2 2 2
  spline S376 degree 2 poles (-7.2911, -18.1566) (-7.2911, -17.7324) (-6.7893, -17.1999) (-6.417, -17.1999) knots 0 0 0 1 2 2 2
  spline S377 degree 2 poles (-6.417, -17.1999) (-6.0447, -17.1999) (-5.6394, -17.6783) (-5.6394, -18.1024) knots 0 0 0 1 2 2 2
  line L439 (-5.6394, -18.1024) -> (-5.6394, -18.2602)
  spline S378 degree 2 poles (-6.0353, -17.9704) (-6.0376, -17.7489) (-6.2426, -17.5039) (-6.4241, -17.5039) knots 0 0 0 1 2 2 2
  spline S379 degree 2 poles (-6.4241, -17.5039) (-6.6008, -17.5039) (-6.8458, -17.7607) (-6.8741, -17.9704) knots 0 0 0 1 2 2 2
  line L440 (-6.8741, -17.9704) -> (-6.0353, -17.9704)
  spline S380 degree 2 poles (-4.1951, -17.6335) (-4.2681, -17.5746) (-4.4095, -17.5746) knots 0 0 0 1 1 1
  spline S381 degree 2 poles (-4.4095, -17.5746) (-4.5909, -17.5746) (-4.836, -17.9045) (-4.836, -18.1872) knots 0 0 0 1 2 2 2
  line L441 (-4.836, -18.1872) -> (-4.836, -19.0566)
  line L442 (-4.836, -19.0566) -> (-5.246, -19.0566)
  line L443 (-5.246, -19.0566) -> (-5.246, -17.2424)
  line L444 (-5.246, -17.2424) -> (-4.836, -17.2424)
  line L445 (-4.836, -17.2424) -> (-4.836, -17.6146)
  line L446 (-4.836, -17.6146) -> (-4.8289, -17.6146)
  spline S382 degree 2 poles (-4.8289, -17.6146) (-4.7676, -17.4238) (-4.5179, -17.2094) (-4.3647, -17.2094) knots 0 0 0 1 2 2 2
  spline S383 degree 2 poles (-4.3647, -17.2094) (-4.254, -17.2094) (-4.1951, -17.2424) knots 0 0 0 1 1 1
  line L447 (-4.1951, -17.2424) -> (-4.1951, -17.6335)
  spline S384 degree 2 poles (-3.0994, -19.0991) (-3.5188, -19.0991) (-4.0207, -18.5901) (-4.0207, -18.1707) knots 0 0 0 1 2 2 2
  spline S385 degree 2 poles (-4.0207, -18.1707) (-4.0207, -17.7136) (-3.4976, -17.1999) (-3.0547, -17.1999) knots 0 0 0 1 2 2 2
  spline S386 degree 2 poles (-3.0547, -17.1999) (-2.6306, -17.1999) (-2.1546, -17.6995) (-2.1546, -18.1424) knots 0 0 0 1 2 2 2
  spline S387 degree 2 poles (-2.1546, -18.1424) (-2.1546, -18.576) (-2.6683, -19.0991) (-3.0994, -19.0991) knots 0 0 0 1 2 2 2
  spline S388 degree 2 poles (-3.0806, -17.5275) (-3.3209, -17.5275) (-3.6013, -17.8644) (-3.6013, -18.1613) knots 0 0 0 1 2 2 2
  spline S389 degree 2 poles (-3.6013, -18.1613) (-3.6013, -18.4464) (-3.3186, -18.7739) (-3.0806, -18.7739) knots 0 0 0 1 2 2 2
  spline S390 degree 2 poles (-3.0806, -18.7739) (-2.8379, -18.7739) (-2.5764, -18.4511) (-2.5764, -18.1542) knots 0 0 0 1 2 2 2
  spline S391 degree 2 poles (-2.5764, -18.1542) (-2.5764, -17.8526) (-2.8379, -17.5275) (-3.0806, -17.5275) knots 0 0 0 1 2 2 2
  line L448 (-0.3427, -19.0566) -> (-0.7432, -19.0566)
  line L449 (-0.7432, -19.0566) -> (-0.7432, -18.7739)
  line L450 (-0.7432, -18.7739) -> (-0.7503, -18.7739)
  spline S392 degree 2 poles (-0.7503, -18.7739) (-0.9364, -19.0991) (-1.2993, -19.0991) knots 0 0 0 1 1 1
  spline S393 degree 2 poles (-1.2993, -19.0991) (-1.5679, -19.0991) (-1.8719, -18.8092) (-1.8719, -18.5689) knots 0 0 0 1 2 2 2
  spline S394 degree 2 poles (-1.8719, -18.5689) (-1.8719, -18.0553) (-1.2781, -17.9704) knots 0 0 0 1 1 1
  line L451 (-1.2781, -17.9704) -> (-0.7409, -17.895)
  spline S395 degree 2 poles (-0.7409, -17.895) (-0.7409, -17.5063) (-1.1084, -17.5063) knots 0 0 0 1 1 1
  spline S396 degree 2 poles (-1.1084, -17.5063) (-1.4336, -17.5063) (-1.6928, -17.7301) knots 0 0 0 1 1 1
  line L452 (-1.6928, -17.7301) -> (-1.6928, -17.3696)
  spline S397 degree 2 poles (-1.6928, -17.3696) (-1.4077, -17.1999) (-1.0307, -17.1999) knots 0 0 0 1 1 1
  spline S398 degree 2 poles (-1.0307, -17.1999) (-0.3427, -17.1999) (-0.3427, -17.8762) knots 0 0 0 1 1 1
  line L453 (-0.3427, -17.8762) -> (-0.3427, -19.0566)
  line L454 (-0.7409, -18.166) -> (-1.1226, -18.2202)
  spline S399 degree 2 poles (-1.1226, -18.2202) (-1.2993, -18.2414) (-1.4784, -18.3686) (-1.4784, -18.5265) knots 0 0 0 1 2 2 2
  spline S400 degree 2 poles (-1.4784, -18.5265) (-1.4784, -18.6419) (-1.3134, -18.788) (-1.1744, -18.788) knots 0 0 0 1 2 2 2
  spline S401 degree 2 poles (-1.1744, -18.788) (-0.9859, -18.788) (-0.7409, -18.5241) (-0.7409, -18.3239) knots 0 0 0 1 2 2 2
  line L455 (-0.7409, -18.3239) -> (-0.7409, -18.166)
  line L456 (-18.8178, -21.3336) -> (-18.8178, -23.9302)
  line L457 (-18.8178, -23.9302) -> (-19.2277, -23.9302)
  line L458 (-19.2277, -23.9302) -> (-19.2277, -21.8379)
  spline S402 degree 2 poles (-19.2277, -21.8379) (-19.3385, -21.918) (-19.5953, -22.0287) (-19.7602, -22.0711) knots 0 0 0 1 2 2 2
  line L459 (-19.7602, -22.0711) -> (-19.7602, -21.7201)
  spline S403 degree 2 poles (-19.7602, -21.7201) (-19.6589, -21.6871) (-19.4681, -21.6117) (-19.2819, -21.5198) (-19.0911, -21.4067) (-18.9898, -21.3336) knots 0 0 0 1 2 3 4 4 4
  line L460 (-18.9898, -21.3336) -> (-18.8178, -21.3336)
  spline S404 degree 2 poles (-16.5581, -23.1149) (-16.5581, -23.3058) (-16.6854, -23.6215) (-16.9069, -23.8501) (-17.2132, -23.975) (-17.3922, -23.975) knots 0 0 0 1 2 3 4 4 4
  spline S405 degree 2 poles (-17.3922, -23.975) (-17.5855, -23.975) (-17.9059, -23.8265) (-18.1368, -23.532) (-18.264, -23.0937) (-18.264, -22.8063) knots 0 0 0 1 2 3 4 4 4
  spline S406 degree 2 poles (-18.264, -22.8063) (-18.264, -22.4528) (-18.0968, -21.9086) (-17.8022, -21.5386) (-17.4064, -21.3478) (-17.1755, -21.3478) knots 0 0 0 1 2 3 4 4 4
  spline S407 degree 2 poles (-17.1755, -21.3478) (-17.0317, -21.3478) (-16.7961, -21.3878) (-16.7254, -21.4208) knots 0 0 0 1 2 2 2
  line L461 (-16.7254, -21.4208) -> (-16.7254, -21.7907)
  spline S408 degree 2 poles (-16.7254, -21.7907) (-16.815, -21.7436) (-17.02, -21.68) (-17.1543, -21.68) knots 0 0 0 1 2 2 2
  spline S409 degree 2 poles (-17.1543, -21.68) (-17.3027, -21.68) (-17.5548, -21.8002) (-17.7362, -22.0334) (-17.8423, -22.3751) (-17.8423, -22.5989) knots 0 0 0 1 2 3 4 4 4
  line L462 (-17.8423, -22.5989) -> (-17.8329, -22.5989)
  spline S410 degree 2 poles (-17.8329, -22.5989) (-17.7504, -22.474) (-17.4724, -22.328) (-17.2839, -22.328) knots 0 0 0 1 2 2 2
  spline S411 degree 2 poles (-17.2839, -22.328) (-17.1189, -22.328) (-16.8503, -22.4363) (-16.6618, -22.639) (-16.5581, -22.9311) (-16.5581, -23.1149) knots 0 0 0 1 2 3 4 4 4
  spline S412 degree 2 poles (-16.9728, -23.1479) (-16.9728, -23.0372) (-17.0247, -22.8581) (-17.1283, -22.7285) (-17.2862, -22.6578) (-17.3922, -22.6578) knots 0 0 0 1 2 3 4 4 4
  spline S413 degree 2 poles (-17.3922, -22.6578) (-17.4983, -22.6578) (-17.6609, -22.7332) (-17.7692, -22.8581) (-17.8258, -23.016) (-17.8258, -23.1008) knots 0 0 0 1 2 3 4 4 4
  spline S414 degree 2 poles (-17.8258, -23.1008) (-17.8258, -23.1903) (-17.7739, -23.3788) (-17.6679, -23.5343) (-17.503, -23.6357) (-17.3899, -23.6357) knots 0 0 0 1 2 3 4 4 4
  spline S415 degree 2 poles (-17.3899, -23.6357) (-17.2886, -23.6357) (-17.1331, -23.5603) (-17.027, -23.4307) (-16.9728, -23.2516) (-16.9728, -23.1479) knots 0 0 0 1 2 3 4 4 4
  line L463 (-15.3329, -21.3336) -> (-15.3329, -23.9302)
  line L464 (-15.3329, -23.9302) -> (-15.7429, -23.9302)
  line L465 (-15.7429, -23.9302) -> (-15.7429, -21.8379)
  spline S416 degree 2 poles (-15.7429, -21.8379) (-15.8536, -21.918) (-16.1105, -22.0287) (-16.2754, -22.0711) knots 0 0 0 1 2 2 2
  line L466 (-16.2754, -22.0711) -> (-16.2754, -21.7201)
  spline S417 degree 2 poles (-16.2754, -21.7201) (-16.1741, -21.6871) (-15.9832, -21.6117) (-15.7971, -21.5198) (-15.6062, -21.4067) (-15.5049, -21.3336) knots 0 0 0 1 2 3 4 4 4
  line L467 (-15.5049, -21.3336) -> (-15.3329, -21.3336)
  spline S418 degree 2 poles (-13.0733, -23.1149) (-13.0733, -23.3058) (-13.2005, -23.6215) (-13.422, -23.8501) (-13.7283, -23.975) (-13.9074, -23.975) knots 0 0 0 1 2 3 4 4 4
  spline S419 degree 2 poles (-13.9074, -23.975) (-14.1006, -23.975) (-14.4211, -23.8265) (-14.652, -23.532) (-14.7792, -23.0937) (-14.7792, -22.8063) knots 0 0 0 1 2 3 4 4 4
  spline S420 degree 2 poles (-14.7792, -22.8063) (-14.7792, -22.4528) (-14.6119, -21.9086) (-14.3174, -21.5386) (-13.9215, -21.3478) (-13.6906, -21.3478) knots 0 0 0 1 2 3 4 4 4
  spline S421 degree 2 poles (-13.6906, -21.3478) (-13.5469, -21.3478) (-13.3113, -21.3878) (-13.2406, -21.4208) knots 0 0 0 1 2 2 2
  line L468 (-13.2406, -21.4208) -> (-13.2406, -21.7907)
  spline S422 degree 2 poles (-13.2406, -21.7907) (-13.3301, -21.7436) (-13.5351, -21.68) (-13.6694, -21.68) knots 0 0 0 1 2 2 2
  spline S423 degree 2 poles (-13.6694, -21.68) (-13.8179, -21.68) (-14.07, -21.8002) (-14.2514, -22.0334) (-14.3574, -22.3751) (-14.3574, -22.5989) knots 0 0 0 1 2 3 4 4 4
  line L469 (-14.3574, -22.5989) -> (-14.348, -22.5989)
  spline S424 degree 2 poles (-14.348, -22.5989) (-14.2655, -22.474) (-13.9875, -22.328) (-13.799, -22.328) knots 0 0 0 1 2 2 2
  spline S425 degree 2 poles (-13.799, -22.328) (-13.6341, -22.328) (-13.3655, -22.4363) (-13.177, -22.639) (-13.0733, -22.9311) (-13.0733, -23.1149) knots 0 0 0 1 2 3 4 4 4
  spline S426 degree 2 poles (-13.488, -23.1479) (-13.488, -23.0372) (-13.5398, -22.8581) (-13.6435, -22.7285) (-13.8014, -22.6578) (-13.9074, -22.6578) knots 0 0 0 1 2 3 4 4 4
  spline S427 degree 2 poles (-13.9074, -22.6578) (-14.0134, -22.6578) (-14.176, -22.7332) (-14.2844, -22.8581) (-14.3409, -23.016) (-14.3409, -23.1008) knots 0 0 0 1 2 3 4 4 4
  spline S428 degree 2 poles (-14.3409, -23.1008) (-14.3409, -23.1903) (-14.2891, -23.3788) (-14.1831, -23.5343) (-14.0181, -23.6357) (-13.905, -23.6357) knots 0 0 0 1 2 3 4 4 4
  spline S429 degree 2 poles (-13.905, -23.6357) (-13.8037, -23.6357) (-13.6482, -23.5603) (-13.5422, -23.4307) (-13.488, -23.2516) (-13.488, -23.1479) knots 0 0 0 1 2 3 4 4 4
  spline S430 degree 2 poles (-11.1153, -21.5952) (-11.2755, -21.8873) (-11.5583, -22.4599) (-11.7892, -23.0372) (-11.9588, -23.6239) (-12.0036, -23.9302) knots 0 0 0 1 2 3 4 4 4
  line L470 (-12.0036, -23.9302) -> (-12.4348, -23.9302)
  spline S431 degree 2 poles (-12.4348, -23.9302) (-12.3924, -23.6569) (-12.2345, -23.1126) (-12.0224, -22.5706) (-11.7585, -22.0217) (-11.6101, -21.7413) knots 0 0 0 1 2 3 4 4 4
  line L471 (-11.6101, -21.7413) -> (-12.8118, -21.7413)
  line L472 (-12.8118, -21.7413) -> (-12.8118, -21.3902)
  line L473 (-12.8118, -21.3902) -> (-11.1153, -21.3902)
  line L474 (-11.1153, -21.3902) -> (-11.1153, -21.5952)
  spline S432 degree 2 poles (-10.8302, -23.221) (-10.8302, -23.1126) (-10.7736, -22.9076) (-10.6652, -22.7332) (-10.498, -22.5966) (-10.3872, -22.5542) knots 0 0 0 1 2 3 4 4 4
  spline S433 degree 2 poles (-10.3872, -22.5542) (-10.5521, -22.4599) (-10.7454, -22.1724) (-10.7454, -21.9957) knots 0 0 0 1 2 2 2
  spline S434 degree 2 poles (-10.7454, -21.9957) (-10.7454, -21.8567) (-10.6299, -21.6187) (-10.4273, -21.4444) (-10.1516, -21.3478) (-9.9867, -21.3478) knots 0 0 0 1 2 3 4 4 4
  spline S435 degree 2 poles (-9.9867, -21.3478) (-9.8217, -21.3478) (-9.5437, -21.4467) (-9.3411, -21.6211) (-9.228, -21.8591) (-9.228, -21.9957) knots 0 0 0 1 2 3 4 4 4
  spline S436 degree 2 poles (-9.228, -21.9957) (-9.228, -22.1724) (-9.4235, -22.4599) (-9.5837, -22.5542) knots 0 0 0 1 2 2 2
  spline S437 degree 2 poles (-9.5837, -22.5542) (-9.473, -22.5966) (-9.3057, -22.7309) (-9.1926, -22.9052) (-9.1361, -23.1102) (-9.1361, -23.221) knots 0 0 0 1 2 3 4 4 4
  spline S438 degree 2 poles (-9.1361, -23.221) (-9.1361, -23.3883) (-9.2586, -23.6639) (-9.4824, -23.8595) (-9.7934, -23.9702) (-9.9819, -23.9702) knots 0 0 0 1 2 3 4 4 4
  spline S439 degree 2 poles (-9.9819, -23.9702) (-10.1681, -23.9702) (-10.4791, -23.8595) (-10.7029, -23.6639) (-10.8302, -23.3883) (-10.8302, -23.221) knots 0 0 0 1 2 3 4 4 4
  spline S440 degree 2 poles (-10.4296, -23.188) (-10.4296, -23.294) (-10.366, -23.4684) (-10.2482, -23.5885) (-10.0833, -23.6522) (-9.9819, -23.6522) knots 0 0 0 1 2 3 4 4 4
  spline S441 degree 2 poles (-9.9819, -23.6522) (-9.8853, -23.6522) (-9.7228, -23.5862) (-9.6026, -23.4637) (-9.5366, -23.294) (-9.5366, -23.188) knots 0 0 0 1 2 3 4 4 4
  spline S442 degree 2 poles (-9.5366, -23.188) (-9.5366, -23.089) (-9.6002, -22.9194) (-9.7157, -22.7921) (-9.8806, -22.7167) (-9.9819, -22.7167) knots 0 0 0 1 2 3 4 4 4
  spline S443 degree 2 poles (-9.9819, -22.7167) (-10.0786, -22.7167) (-10.2435, -22.7851) (-10.3613, -22.9123) (-10.4296, -23.0843) (-10.4296, -23.188) knots 0 0 0 1 2 3 4 4 4
  spline S444 degree 2 poles (-10.3424, -22.0381) (-10.3424, -22.1183) (-10.2859, -22.2549) (-10.1893, -22.3562) (-10.0597, -22.4128) (-9.9867, -22.4128) knots 0 0 0 1 2 3 4 4 4
  spline S445 degree 2 poles (-9.9867, -22.4128) (-9.9113, -22.4128) (-9.7817, -22.3539) (-9.6851, -22.2526) (-9.6285, -22.1183) (-9.6285, -22.0381) knots 0 0 0 1 2 3 4 4 4
  spline S446 degree 2 poles (-9.6285, -22.0381) (-9.6285, -21.9604) (-9.6827, -21.8214) (-9.7793, -21.7224) (-9.9089, -21.6659) (-9.9867, -21.6659) knots 0 0 0 1 2 3 4 4 4
  spline S447 degree 2 poles (-9.9867, -21.6659) (-10.0644, -21.6659) (-10.1964, -21.7248) (-10.2906, -21.8261) (-10.3424, -21.9627) (-10.3424, -22.0381) knots 0 0 0 1 2 3 4 4 4
  line L475 (-27.9268, -70.1764) -> (-26.886, -70.1764)
  spline S448 degree 2 poles (-26.886, -70.1764) (-25.8272, -70.1764) (-25.8272, -70.9925) knots 0 0 0 1 1 1
  spline S449 degree 2 poles (-25.8272, -70.9925) (-25.8272, -71.3101) (-26.0157, -71.5219) knots 0 0 0 1 1 1
  spline S450 degree 2 poles (-26.0157, -71.5219) (-26.1888, -71.713) (-26.4548, -71.7698) knots 0 0 0 1 1 1
  line L476 (-26.4548, -71.7698) -> (-25.7446, -73.2264)
  line L477 (-25.7446, -73.2264) -> (-26.2017, -73.2264)
  line L478 (-26.2017, -73.2264) -> (-26.8551, -71.8396)
  line L479 (-26.8551, -71.8396) -> (-27.5033, -71.8396)
  line L480 (-27.5033, -71.8396) -> (-27.5033, -73.2264)
  line L481 (-27.5033, -73.2264) -> (-27.9268, -73.2264)
  line L482 (-27.9268, -73.2264) -> (-27.9268, -70.1764)
  line L483 (-27.5033, -70.538) -> (-27.5033, -71.4858)
  line L484 (-27.5033, -71.4858) -> (-26.9325, -71.4858)
  spline S451 degree 2 poles (-26.9325, -71.4858) (-26.2662, -71.4858) (-26.2662, -70.9977) knots 0 0 0 1 1 1
  spline S452 degree 2 poles (-26.2662, -70.9977) (-26.2662, -70.7497) (-26.4264, -70.6438) knots 0 0 0 1 1 1
  spline S453 degree 2 poles (-26.4264, -70.6438) (-26.5813, -70.538) (-26.9067, -70.538) knots 0 0 0 1 1 1
  line L485 (-26.9067, -70.538) -> (-27.5033, -70.538)
  line L486 (-23.2705, -70.1764) -> (-23.2705, -70.5509)
  line L487 (-23.2705, -70.5509) -> (-24.789, -70.5509)
  line L488 (-24.789, -70.5509) -> (-24.789, -71.4212)
  line L489 (-24.789, -71.4212) -> (-23.6398, -71.4212)
  line L490 (-23.6398, -71.4212) -> (-23.6398, -71.7957)
  line L491 (-23.6398, -71.7957) -> (-24.789, -71.7957)
  line L492 (-24.789, -71.7957) -> (-24.789, -72.8519)
  line L493 (-24.789, -72.8519) -> (-23.2421, -72.8519)
  line L494 (-23.2421, -72.8519) -> (-23.2421, -73.2264)
  line L495 (-23.2421, -73.2264) -> (-25.2203, -73.2264)